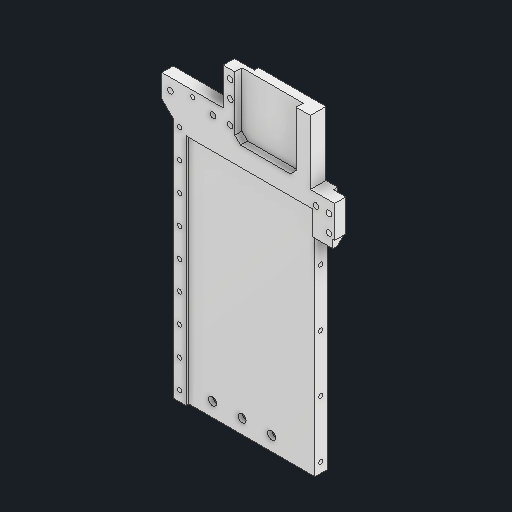
# Autodesk Inventor part: BottomSlideMount
Saved by Autodesk Inventor 2026.2 (Build 302298000, 298)
## iProperties
Created: 2026-01-21
Part Number: BottomSlideMount
Material: ABS Plastic
Document SubType Name: Modeling
Designer: gaoet
Density: 1.06 g/cm^3
Appearance: Smooth - White
Author: gaoet
Autodesk Inventor part; units mm, degrees
ref_plane "YZ Plane" through (0, 0, 0) normal (1, 0, 0) x (0, 1, 0)
ref_plane "XZ Plane" through (0, 0, 0) normal (0, 1, 0) x (-1, 0, 0)
ref_plane "XY Plane" through (0, 0, 0) normal (0, 0, 1) x (1, 0, 0)
sketch "Sketch1" plane through (0, 0, 0) normal (0, 0, 1) x (1, 0, 0)
  line L0 (-117.5, -110) -> (117.5, -110)
  line L1 (117.5, -110) -> (117.5, 110)
  line L2 (117.5, 110) -> (-117.5, 110)
  line L3 (-117.5, 110) -> (-117.5, -110)
  line L4 (-117.5, -110) -> (117.5, 110) construction
  line L5 (117.5, -110) -> (-117.5, 110) construction
  line L6 (0, 110) -> (0, -110) construction
  line L7 (-4, -110) -> (4, -110) construction
  line L8 (4, -110) -> (4, 110) construction
  line L9 (4, 110) -> (-4, 110) construction
  line L10 (-4, 110) -> (-4, -110) construction
  line L11 (-4, -110) -> (4, 110) construction
  line L12 (4, -110) -> (-4, 110) construction
  line L13 (-12, -110) -> (12, -110) construction
  line L14 (12, -110) -> (12, 110) construction
  line L15 (12, 110) -> (-12, 110) construction
  line L16 (-12, 110) -> (-12, -110) construction
  line L17 (-12, -110) -> (12, 110) construction
  line L18 (12, -110) -> (-12, 110) construction
  line L19 (-13, -110) -> (13, -110)
  line L20 (13, -110) -> (13, 110)
  line L21 (13, 110) -> (-13, 110)
  line L22 (-13, 110) -> (-13, -110)
  line L23 (-13, -110) -> (13, 110) construction
  line L24 (13, -110) -> (-13, 110) construction
  point P0 (0, 0)
  point P1 (-13, -110)
  point P2 (-13, 110)
  dimension "d0" = 235
  dimension "d1" = 220
  dimension "d4" = 8
  dimension "d5" = 24
  dimension "d6" = 26
  constraints: 50 end point, 10 midpoint, 8 parallel, 4 horizontal, 4 perpendicular, 3 point on line
  measures "d0" distance of L2.end L1.end
  measures "d1" distance of L1.end L0.end
  measures "d4" distance of L9.end L8.end
  measures "d5" distance of L15.end L14.end
  measures "d6" distance of L21.end L20.end
extrude "Extrusion1" add sketch "Sketch1" along normal blind 8 contours L3 L2 L22 L0
sketch "Sketch2" plane through (0, 0, 8) normal (0, 0, 1) x (1, 0, 0)
  line L0 (-13, 110) -> (-117.5, 110) projected
  line L1 (-13, -110) -> (-13, 110) projected
  point P0 (0, 0)
  point P1 (-17.25, 102)
  point P2 (-17.25, 90)
  dimension "d7" = 8
  dimension "d8" = 12
  dimension "d9" = 4.25
  constraints: 1 vertical alignment
  measures "d7" distance from line of L0 point (-17.25, 102)
  measures "d8" distance of point (-17.25, 90) point (-17.25, 102)
  measures "d9" distance from line of L1 point (-17.25, 90)
hole "Hole1" at (-17.25, 102, 8) direction (0, 0, -1) diameter 4 end through all
sketch "Sketch3" plane through (0, 0, 8) normal (0, 0, 1) x (1, 0, 0)
  line L0 (-117.5, -110) -> (-13, -110) projected
  line L1 (-13, -110) -> (-13, 110) projected
  line L2 (-13, 110) -> (-117.5, 110) projected
  line L3 (-117.5, 110) -> (-117.5, -110) projected
  line L4 (-13, 110) -> (-4.25, 110)
  line L5 (-4.25, 110) -> (-4.25, 82)
  line L6 (-4.25, 82) -> (-13, 82)
  line L7 (-13, 82) -> (-13, 110)
  point P0 (0, 0)
  point P1 (-13, 82)
  dimension "d17" = 8.75
  dimension "d18" = 28
  constraints: 8 end point, 2 parallel, 1 horizontal, 1 perpendicular
  measures "d17" distance of L5.end L6.end
  measures "d18" distance of L4.end L5.end
extrude "Extrusion2" add sketch "Sketch3" against normal up to surface (8 mm away) contours L1 L4 L5 L6
sketch "Sketch4" plane through (0, 0, 8) normal (0, 0, 1) x (1, 0, 0)
  circle A0 centre (-17.25, 102) radius 2 projected
  line L0 (-117.5, -110) -> (-13, -110) projected
  line L1 (-13, -110) -> (-13, 82) projected
  line L2 (-13, 82) -> (-4.25, 82) projected
  line L3 (-4.25, 82) -> (-4.25, 110) projected
  line L4 (-4.25, 110) -> (-117.5, 110) projected
  line L5 (-117.5, 110) -> (-117.5, -110) projected
  point P0 (0, 0)
  point P1 (-8.25, 102)
  point P2 (-8.25, 90)
  dimension "d21" = 4
  constraints: 1 horizontal alignment, 1 vertical alignment
  measures "d21" distance from line of L3 point (-8.25, 102)
hole "Hole2" at (-8.25, 102, 8) at (-8.25, 90, 8) direction (0, 0, -1) diameter 4 end through all
sketch "Sketch5" plane through (0, 0, 8) normal (0, 0, 1) x (1, 0, 0)
  circle A0 centre (-8.25, 90) radius 2 projected
  circle A1 centre (-8.25, 102) radius 2 projected
  circle A2 centre (-17.25, 102) radius 2 projected
  line L0 (-117.5, -110) -> (-13, -110) projected
  line L1 (-13, -110) -> (-13, 82) projected
  line L2 (-13, 82) -> (-4.25, 82) projected
  line L3 (-4.25, 82) -> (-4.25, 110) projected
  line L4 (-4.25, 110) -> (-117.5, 110) projected
  line L5 (-117.5, 110) -> (-117.5, -110) projected
  line L6 (-5.375, 82) -> (-5.375, 87.5)
  line L7 (-5.375, 87.5) -> (-4.25, 87.5)
  point P0 (0, 0)
  dimension "d29" = 5.5
  dimension "d30" = 1.125
  constraints: 4 end point, 2 point on line, 1 horizontal, 1 perpendicular
  measures "d29" distance of L6.start L6.end
  measures "d30" distance of L6.end L7.end
extrude "Extrusion3" cut sketch "Sketch5" against normal blind 10 contours L6 L7 L3 L2
sketch "Sketch6" plane through (-117.5, -110, 0) normal (0, -1, 0) x (1, 0, 0)
  line L0 (0, 0) -> (104.5, 0) projected
  line L1 (104.5, 0) -> (104.5, 8) projected
  line L2 (0, 8) -> (104.5, 8) projected
  line L3 (0, 0) -> (0, 8) projected
  line L4 (0, 0) -> (0, 8) projected
  line L5 (0, 5) -> (15.25, 5)
  line L6 (15.25, 5) -> (15.25, 0)
  line L7 (9, 5) -> (9, 3.5)
  line L8 (9, 3.5) -> (15.25, 3.5)
  point P0 (117.5, 0)
  point P1 (0, 4)
  dimension "d33" = 15.25
  dimension "d34" = 5
  dimension "d35" = 9
  dimension "d36" = 1.5
  constraints: 8 end point, 4 point on line, 2 perpendicular, 1 horizontal, 1 midpoint, 1 vertical
  measures "d33" distance of L5.start L5.end
  measures "d34" distance of L5.end L6.end
  measures "d35" distance from line of point (0, 4) L7
  measures "d36" distance between parallel lines of L5 L8
extrude "Extrusion4" cut sketch "Sketch6" against normal through all contours L3 L5 L7 L8 L6 L0
chamfer "Chamfer1" distance 5 angle 45 1 edges at (-9.1875, 82, 0)
sketch "Sketch7" plane through (0, 0, 8) normal (0, 0, 1) x (1, 0, 0)
  line L0 (-117.5, -65) -> (-13, -65)
  line L1 (-5.375, 87.5) -> (-4.25, 87.5) projected
  line L2 (-4.25, 87.5) -> (-4.25, 110) projected
  line L3 (-4.25, 110) -> (-117.5, 110) projected
  line L4 (-117.5, 110) -> (-117.5, -110) projected
  line L5 (-117.5, -110) -> (-13, -110) projected
  line L6 (-13, -110) -> (-13, 82) projected
  line L7 (-13, 82) -> (-5.375, 82) projected
  line L8 (-5.375, 82) -> (-5.375, 87.5) projected
  circle A0 centre (-8.25, 90) radius 2 projected
  circle A1 centre (-8.25, 102) radius 2 projected
  circle A2 centre (-17.25, 102) radius 2 projected
  point P0 (0, 0)
  dimension "d42" = 45
  constraints: 2 end point, 2 point on line, 1 horizontal, 1 perpendicular
  measures "d42" distance between parallel lines of L5 L0
extrude "Extrusion5" cut sketch "Sketch7" against normal blind 10 contours L0 L6 L5 L4
sketch "Sketch8" plane through (-117.5, 110, 8) normal (0, 1, 0) x (1, 0, 0)
  line L0 (113.25, 0) -> (0, 0) projected
  line L1 (15.25, 8) -> (15.25, 4.5) projected
  line L2 (15.25, 4.5) -> (9, 4.5) projected
  line L3 (9, 4.5) -> (9, 3) projected
  line L4 (9, 3) -> (0, 3) projected
  line L5 (0, 3) -> (0, 0) projected
  line L6 (113.25, 0) -> (0, 0) projected
  line L7 (113.25, 0) -> (113.25, 8) projected
  line L8 (15.25, 8) -> (113.25, 8) projected
  line L9 (96.25, 0) -> (96.25, 8)
  line L10 (15.25, 8) -> (0, 8)
  line L11 (0, 8) -> (0, 3)
  point P0 (117.5, 8)
  point P1 (96.25, 4)
  dimension "d45" = 96.25
  constraints: 6 end point, 2 perpendicular, 2 point on line, 1 horizontal, 1 midpoint
  measures "d45" horizontal distance of L4.end point (96.25, 4)
extrude "Extrusion6" add sketch "Sketch8" along normal blind 45 contours L0 L5 L4 L3 L2 L1 L8 L9 | L11 L10 L1 L2 L3 L4
sketch "Sketch9" plane through (0, 0, 0) normal (0, 0, -1) x (-1, 0, 0)
  line L0 (13, -65) -> (102.25, -65) projected
  line L1 (102.25, -65) -> (102.25, 110) projected
  line L2 (102.25, 110) -> (117.5, 110) projected
  line L3 (117.5, 110) -> (117.5, 155) projected
  line L4 (21.25, 155) -> (117.5, 155) projected
  line L5 (21.25, 110) -> (21.25, 155) projected
  line L6 (21.25, 110) -> (4.25, 110) projected
  line L7 (4.25, 110) -> (4.25, 87.5) projected
  line L8 (4.25, 87.5) -> (5.375, 87.5) projected
  line L9 (5.375, 87.5) -> (5.375, 87) projected
  line L10 (13, 87) -> (5.375, 87) projected
  line L11 (13, -65) -> (13, 87) projected
  circle A0 centre (8.25, 90) radius 2 projected
  circle A1 centre (8.25, 102) radius 2 projected
  circle A2 centre (17.25, 102) radius 2 projected
  line L12 (82.5, 155) -> (82.5, 129)
  line L13 (82.5, 129) -> (117.5, 129)
  line L14 (21.25, 155) -> (117.5, 155) projected
  point P0 (0, 0)
  dimension "d49" = 35
  dimension "d50" = 26
  constraints: 4 end point, 2 point on line, 1 perpendicular, 1 vertical
  measures "d49" distance of L12.end L13.end
  measures "d50" distance of L12.start L12.end
extrude "Extrusion7" cut sketch "Sketch9" against normal through all contours L13 L12 L4 L3
sketch "Sketch10" plane through (0, 0, 0) normal (0, 0, -1) x (-1, 0, 0)
  line L0 (21.25, 155) -> (82.5, 155) projected
  line L1 (82.5, 129) -> (82.5, 155) projected
  point P0 (0, 0)
  point P1 (77.5, 149)
  point P2 (77.5, 137)
  point P3 (77.5, 121)
  point P4 (89.5, 121)
  point P5 (119.5, 121)
  dimension "d53" = 12
  dimension "d54" = 6
  dimension "d55" = 16
  dimension "d56" = 5
  dimension "d57" = 12
  dimension "d58" = 30
  constraints: 2 horizontal alignment, 2 vertical alignment
  measures "d53" distance of point (77.5, 149) point (77.5, 137)
  measures "d54" distance from line of L0 point (77.5, 149)
  measures "d55" distance of point (77.5, 137) point (77.5, 121)
  measures "d56" distance from line of point (77.5, 149) L1
  measures "d57" distance of point (89.5, 121) point (77.5, 121)
  measures "d58" distance of point (89.5, 121) point (119.5, 121)
sketch "Sketch11" plane through (-117.5, 110, 8) normal (0, -1, 0) x (1, 0, 0)
  line L0 (15.25, -8) -> (15.25, -4.5) projected
  line L1 (15.25, -4.5) -> (9, -4.5) projected
  line L2 (9, -4.5) -> (9, -3) projected
  line L3 (9, -3) -> (0, -3) projected
  line L4 (0, -8) -> (0, -3) projected
  line L5 (15.25, -8) -> (0, -8) projected
  point P0 (117.5, -8)
extrude "Extrusion8" add sketch "Sketch11" along normal blind 26
sketch "Sketch12" plane through (0, 0, 0) normal (0, 0, -1) x (-1, 0, 0)
  line L0 (82.5, 129) -> (82.5, 155) projected
  line L1 (21.25, 155) -> (82.5, 155) projected
  line L2 (21.25, 110) -> (21.25, 155) projected
  line L3 (21.25, 110) -> (4.25, 110) projected
  line L4 (4.25, 110) -> (4.25, 87.5) projected
  line L5 (4.25, 87.5) -> (5.375, 87.5) projected
  line L6 (5.375, 87.5) -> (5.375, 87) projected
  line L7 (13, 87) -> (5.375, 87) projected
  line L8 (13, -65) -> (13, 87) projected
  line L9 (13, -65) -> (102.25, -65) projected
  line L10 (102.25, -65) -> (102.25, 84) projected
  line L11 (117.5, 84) -> (102.25, 84) projected
  line L12 (117.5, 129) -> (117.5, 84) projected
  line L13 (117.5, 129) -> (82.5, 129) projected
  circle A0 centre (8.25, 90) radius 2 projected
  circle A1 centre (8.25, 102) radius 2 projected
  circle A2 centre (17.25, 102) radius 2 projected
  line L14 (117.5, 129) -> (125.5, 129)
  line L15 (125.5, 129) -> (125.5, 113)
  line L16 (125.5, 113) -> (117.5, 113)
  point P0 (0, 0)
  point P1 (125.5, 121)
  dimension "d61" = 8
  dimension "d62" = 16
  constraints: 6 end point, 2 horizontal, 1 midpoint, 1 perpendicular, 1 point on line
  measures "d61" distance from line of L12 point (125.5, 121)
  measures "d62" distance of L14.end L15.end
extrude "Extrusion9" add sketch "Sketch12" against normal up to surface (8 mm away) contours L14 L15 L16 L12
chamfer "Chamfer2" distance 8 angle 45 1 edges at (-117.5, 113, 4)
hole "Hole3" at (-77.5, 149, 0) at (-77.5, 137, 0) at (-77.5, 121, 0) at (-89.5, 121, 0) at (-119.5, 121, 0) direction (0, 0, 1) diameter 4 end through all
sketch "Sketch13" plane through (0, 0, 0) normal (0, 0, -1) x (-1, 0, 0)
  line L0 (117.5, 105) -> (117.5, 84) projected
  line L1 (125.5, 129) -> (82.5, 129) projected
  point P0 (0, 0)
  point P1 (103.75, 125)
  dimension "d75" = 13.75
  dimension "d76" = 4
  measures "d75" distance from line of L0 point (103.75, 125)
  measures "d76" distance from line of L1 point (103.75, 125)
hole "Hole4" at (-103.75, 125, 0) direction (0, 0, 1) diameter 3 end through all
sketch "Sketch14" plane through (0, 0, 0) normal (0, 0, -1) x (-1, 0, 0)
  circle A0 centre (103.75, 125) radius 1.5 projected
  circle A1 centre (119.5, 121) radius 2 projected
  circle A2 centre (89.5, 121) radius 2 projected
  circle A3 centre (77.5, 121) radius 2 projected
  circle A4 centre (77.5, 137) radius 2 projected
  circle A5 centre (77.5, 149) radius 2 projected
  line L0 (82.5, 129) -> (82.5, 155) projected
  line L1 (21.25, 155) -> (82.5, 155) projected
  line L2 (21.25, 110) -> (21.25, 155) projected
  line L3 (21.25, 110) -> (4.25, 110) projected
  line L4 (4.25, 110) -> (4.25, 87.5) projected
  line L5 (4.25, 87.5) -> (5.375, 87.5) projected
  line L6 (5.375, 87.5) -> (5.375, 87) projected
  line L7 (13, 87) -> (5.375, 87) projected
  line L8 (13, -65) -> (13, 87) projected
  line L9 (13, -65) -> (102.25, -65) projected
  line L10 (102.25, -65) -> (102.25, 84) projected
  line L11 (117.5, 84) -> (102.25, 84) projected
  line L12 (117.5, 105) -> (117.5, 84) projected
  line L13 (125.5, 113) -> (117.5, 105) projected
  line L14 (125.5, 113) -> (125.5, 129) projected
  line L15 (125.5, 129) -> (82.5, 129) projected
  circle A6 centre (8.25, 90) radius 2 projected
  circle A7 centre (8.25, 102) radius 2 projected
  circle A8 centre (17.25, 102) radius 2 projected
  line L16 (105.3233, 127.725) -> (106.8966, 125)
  line L17 (106.8966, 125) -> (105.3233, 122.275)
  line L18 (105.3233, 122.275) -> (102.1767, 122.275)
  line L19 (102.1767, 122.275) -> (100.6034, 125)
  line L20 (100.6034, 125) -> (102.1767, 127.725)
  line L21 (102.1767, 127.725) -> (105.3233, 127.725)
  point P0 (0, 0)
  point P1 (103.75, 122.275)
  dimension "d84" = 5.45
  constraints: 12 end point, 1 coincident, 1 horizontal, 1 midpoint, 13 other
  measures "d84" distance from line of point (103.75, 122.275) L21
extrude "Extrusion10" cut sketch "Sketch14" against normal blind 2.5 contours L16 L17 L18 L19 L20 L21
sketch "Sketch15" plane through (-117.5, 84, 8) normal (0, -1, 0) x (1, 0, 0)
  line L0 (15.25, -4.5) -> (15.25, -8) projected
  line L1 (9, -4.5) -> (15.25, -4.5) projected
  line L2 (9, -3) -> (9, -4.5) projected
  line L3 (0, -3) -> (9, -3) projected
  line L4 (0, -3) -> (0, -8) projected
  line L5 (0, -8) -> (15.25, -8) projected
  point P0 (117.5, -8)
extrude "Extrusion11" cut sketch "Sketch15" against normal blind 23
sketch "Sketch16" plane through (-108.5, -65, 5) normal (0, 0, -1) x (-1, 0, 0)
  line L0 (9, 172) -> (9, 170) projected
  line L1 (0, 0) -> (0, 172) projected
  line L2 (-6.25, 172) -> (9, 172) projected
  line L3 (9, 170) -> (9, 0) projected
  point P0 (-108.5, 65)
  point P1 (4.5, 167)
  point P2 (4.5, 147)
  point P3 (4.5, 127)
  point P4 (4.5, 107)
  point P5 (4.5, 87)
  point P6 (4.5, 67)
  point P7 (4.5, 47)
  point P8 (4.5, 27)
  point P9 (4.5, 7)
  point P10 (4.5, -13)
  point P11 (4.5, -33)
  dimension "d89" = 9
  dimension "d90" = 5
  dimension "d91" = 4.5
  dimension "d94" = 20
  constraints: 1 vertical, 10 other
  measures "d89" distance between parallel lines of L0 L1
  measures "d90" distance from line of L2 point (4.5, 167)
  measures "d91" distance from line of L3 point (4.5, 167)
  measures "d94" distance of point (4.5, 167) point (4.5, 147)
hole "Hole5" at (-113, 102, 5) at (-113, 82, 5) at (-113, 62, 5) at (-113, 42, 5) at (-113, 22, 5) at (-113, 2, 5) at (-113, -18, 5) at (-113, -38, 5) at (-113, -58, 5) at (-113, -78, 5) at (-113, -98, 5) direction (0, 0, 1) diameter 3 depth 12
sketch "Sketch17" plane through (0, 0, 8) normal (0, 0, 1) x (1, 0, 0)
  circle A0 centre (-113, -58) radius 1.5 projected
  circle A1 centre (-113, -38) radius 1.5 projected
  circle A2 centre (-113, -18) radius 1.5 projected
  circle A3 centre (-113, 2) radius 1.5 projected
  circle A4 centre (-113, 22) radius 1.5 projected
  circle A5 centre (-113, 42) radius 1.5 projected
  circle A6 centre (-113, 62) radius 1.5 projected
  circle A7 centre (-113, 82) radius 1.5 projected
  circle A8 centre (-113, 102) radius 1.5 projected
  circle A9 centre (-103.75, 125) radius 1.5 projected
  circle A10 centre (-119.5, 121) radius 2 projected
  circle A11 centre (-89.5, 121) radius 2 projected
  circle A12 centre (-77.5, 121) radius 2 projected
  circle A13 centre (-77.5, 137) radius 2 projected
  circle A14 centre (-77.5, 149) radius 2 projected
  line L0 (-82.5, 155) -> (-82.5, 129) projected
  line L1 (-82.5, 129) -> (-125.5, 129) projected
  line L2 (-125.5, 113) -> (-125.5, 129) projected
  line L3 (-117.5, 105) -> (-125.5, 113) projected
  line L4 (-117.5, -65) -> (-117.5, 105) projected
  line L5 (-117.5, -65) -> (-13, -65) projected
  line L6 (-13, -65) -> (-13, 82) projected
  line L7 (-13, 82) -> (-5.375, 82) projected
  line L8 (-5.375, 82) -> (-5.375, 87.5) projected
  line L9 (-5.375, 87.5) -> (-4.25, 87.5) projected
  line L10 (-4.25, 87.5) -> (-4.25, 110) projected
  line L11 (-4.25, 110) -> (-21.25, 110) projected
  line L12 (-21.25, 110) -> (-21.25, 155) projected
  line L13 (-82.5, 155) -> (-21.25, 155) projected
  circle A15 centre (-8.25, 90) radius 2 projected
  circle A16 centre (-8.25, 102) radius 2 projected
  circle A17 centre (-17.25, 102) radius 2 projected
  line L14 (-13, 82) -> (-20, 82)
  line L15 (-20, 82) -> (-20, -65)
  line L16 (-20, -65) -> (-13, -65)
  line L17 (-13, -65) -> (-13, 82)
  point P0 (0, 0)
  dimension "d106" = 7
  constraints: 8 end point, 2 parallel, 1 horizontal, 1 perpendicular, 1 point on line
  measures "d106" distance between parallel lines of L6 L15
extrude "Extrusion12" cut sketch "Sketch17" against normal blind 10 contours L15 L14 L6 L5
sketch "Sketch18" plane through (0, 0, 0) normal (0, 0, -1) x (-1, 0, 0)
  circle A0 centre (17.25, 102) radius 2 projected
  circle A1 centre (8.25, 102) radius 2 projected
  circle A2 centre (8.25, 90) radius 2 projected
  circle A3 centre (77.5, 149) radius 2 projected
  circle A4 centre (77.5, 137) radius 2 projected
  circle A5 centre (77.5, 121) radius 2 projected
  circle A6 centre (89.5, 121) radius 2 projected
  circle A7 centre (119.5, 121) radius 2 projected
  line L0 (102.1767, 122.275) -> (100.6034, 125) projected
  line L1 (100.6034, 125) -> (102.1767, 127.725) projected
  line L2 (102.1767, 127.725) -> (105.3233, 127.725) projected
  line L3 (105.3233, 127.725) -> (106.8966, 125) projected
  line L4 (106.8966, 125) -> (105.3233, 122.275) projected
  line L5 (105.3233, 122.275) -> (102.1767, 122.275) projected
  line L6 (13, 82) -> (20, 82) projected
  line L7 (20, 82) -> (20, -65) projected
  line L8 (20, -65) -> (102.25, -65) projected
  line L9 (102.25, -65) -> (102.25, 107) projected
  line L10 (102.25, 107) -> (117.5, 107) projected
  line L11 (117.5, 107) -> (117.5, 105) projected
  line L12 (125.5, 113) -> (117.5, 105) projected
  line L13 (125.5, 113) -> (125.5, 129) projected
  line L14 (125.5, 129) -> (82.5, 129) projected
  line L15 (82.5, 129) -> (82.5, 155) projected
  line L16 (21.25, 155) -> (82.5, 155) projected
  line L17 (21.25, 110) -> (21.25, 155) projected
  line L18 (21.25, 110) -> (4.25, 110) projected
  line L19 (4.25, 110) -> (4.25, 87.5) projected
  line L20 (4.25, 87.5) -> (5.375, 87.5) projected
  line L21 (5.375, 87.5) -> (5.375, 87) projected
  line L22 (13, 87) -> (5.375, 87) projected
  line L23 (13, 82) -> (13, 87) projected
  line L24 (125.5, 155) -> (68.5, 155)
  line L25 (68.5, 155) -> (68.5, 116)
  line L26 (68.5, 116) -> (125.5, 116)
  line L27 (125.5, 116) -> (125.5, 155)
  line L28 (21.25, 155) -> (82.5, 155) projected
  line L29 (125.5, 113) -> (125.5, 129) projected
  line L30 (13, 82) -> (13, 87) projected
  line L31 (13, 87) -> (13, 110)
  point P0 (0, 0)
  point P1 (125.5, 129)
  dimension "d109" = 14
  dimension "d110" = 39
  constraints: 10 end point, 2 collinear, 2 parallel, 1 horizontal, 1 perpendicular, 1 point on line, 1 vertical
  measures "d109" distance between parallel lines of L15 L25
  measures "d110" distance between parallel lines of L16 L26
extrude "Extrusion13" add sketch "Sketch18" along normal blind 3 contours L23 L31 L18 L17 L16 L25 L26 L13 L12 L11 L10 L9 L8 L7 L6
sketch "Sketch19" plane through (-20, -65, 8) normal (1, 0, 0) x (0, 0, -1)
  line L0 (11, 0) -> (0, 0) projected
  line L1 (11, 147) -> (11, 0) projected
  point P0 (8, 65)
  point P1 (6, -33)
  point P2 (6, 7)
  point P3 (6, 47)
  point P4 (6, 127)
  point P5 (6, 87)
  dimension "d113" = 40
  dimension "d114" = 7
  dimension "d115" = 40
  dimension "d116" = 40
  dimension "d117" = 40
  dimension "d118" = 5
  constraints: 4 vertical alignment
  measures "d113" distance of point (6, 7) point (6, -33)
  measures "d114" distance from line of L0 point (6, 7)
  measures "d115" distance of point (6, 47) point (6, 7)
  measures "d116" distance of point (6, 87) point (6, 47)
  measures "d117" distance of point (6, 127) point (6, 87)
  measures "d118" distance from line of L1 point (6, 7)
hole "Hole6" at (-20, -98, 2) at (-20, -58, 2) at (-20, -18, 2) at (-20, 62, 2) at (-20, 22, 2) direction (-1, 0, 0) diameter 3 depth 15
sketch "Sketch20" plane through (0, 0, -3) normal (0, 0, -1) x (-1, 0, 0)
  line L0 (117.5, 105) -> (125.5, 113) projected
  line L1 (125.5, 113) -> (125.5, 116) projected
  line L2 (125.5, 116) -> (68.5, 116) projected
  line L3 (68.5, 116) -> (68.5, 155) projected
  line L4 (68.5, 155) -> (21.25, 155) projected
  line L5 (21.25, 155) -> (21.25, 110) projected
  line L6 (21.25, 110) -> (13, 110) projected
  line L7 (13, 110) -> (13, 82) projected
  line L8 (13, 82) -> (20, 82) projected
  line L9 (20, 82) -> (20, -65) projected
  line L10 (20, -65) -> (102.25, -65) projected
  line L11 (102.25, -65) -> (102.25, 107) projected
  line L12 (102.25, 107) -> (117.5, 107) projected
  line L13 (117.5, 107) -> (117.5, 105) projected
  circle A0 centre (17.25, 102) radius 2 projected
  line L14 (102.25, -45) -> (20, -45)
  line L15 (35, -56.5) -> (35, -59.5) projected
  line L16 (40, -65) -> (40, -45)
  point P0 (0, 0)
  dimension "d126" = 20
  dimension "d127" = 20
  constraints: 4 end point, 4 point on line, 1 horizontal, 1 perpendicular
  measures "d126" distance between parallel lines of L10 L14
  measures "d127" distance between parallel lines of L9 L16
extrude "Extrusion14" cut sketch "Sketch20" against normal blind 3.5 contours L11 L10 L16 L14
chamfer "Chamfer3" distance 10 angle 45 2 edges at (-40, -45, -1.25) (-40, -65, -1.25)
sketch "Sketch21" plane through (0, 0, 8) normal (0, 0, 1) x (1, 0, 0)
  line L0 (-50, -45) -> (-30, -65) projected
  line L1 (-102.25, -65) -> (-30, -65) projected
  line L2 (-102.25, -45) -> (-102.25, -65) projected
  line L3 (-50, -45) -> (-102.25, -45) projected
  point P0 (0, 0)
  point P1 (-91.875, -55)
  point P2 (-71.125, -55)
  point P3 (-50.375, -55)
  point P4 (-102.25, -55)
  dimension "d133" = 20
  dimension "d134" = 20.75
  dimension "d135" = 20.75
  dimension "d136" = 10.375
  dimension "d137" = 10
  constraints: 2 horizontal alignment, 1 midpoint
  measures "d133" distance between parallel lines of L1 L3
  measures "d134" distance of point (-91.875, -55) point (-71.125, -55)
  measures "d135" distance of point (-50.375, -55) point (-71.125, -55)
  measures "d136" distance of point (-102.25, -55) point (-91.875, -55)
  measures "d137" distance from line of L1 point (-91.875, -55)
hole "Hole7" at (-91.875, -55, 8) at (-71.125, -55, 8) at (-50.375, -55, 8) direction (0, 0, -1) diameter 3 depth 15 counterbore diameter 5.75 counterbore depth 5
sketch "Sketch22" plane through (0, 0, 8) normal (0, 0, 1) x (1, 0, 0)
  circle A0 centre (-50.375, -55) radius 2.875 projected
  circle A1 centre (-71.125, -55) radius 2.875 projected
  circle A2 centre (-91.875, -55) radius 2.875 projected
  line L0 (-20, 82) -> (-5.375, 82) projected
  line L1 (-5.375, 82) -> (-5.375, 87.5) projected
  line L2 (-5.375, 87.5) -> (-4.25, 87.5) projected
  line L3 (-4.25, 87.5) -> (-4.25, 110) projected
  line L4 (-4.25, 110) -> (-21.25, 110) projected
  line L5 (-21.25, 110) -> (-21.25, 155) projected
  line L6 (-82.5, 155) -> (-21.25, 155) projected
  line L7 (-82.5, 155) -> (-82.5, 129) projected
  line L8 (-82.5, 129) -> (-125.5, 129) projected
  line L9 (-125.5, 113) -> (-125.5, 129) projected
  line L10 (-117.5, 105) -> (-125.5, 113) projected
  line L11 (-117.5, -65) -> (-117.5, 105) projected
  line L12 (-117.5, -65) -> (-20, -65) projected
  line L13 (-20, -65) -> (-20, 82) projected
  circle A3 centre (-113, -58) radius 1.5 projected
  circle A4 centre (-113, -38) radius 1.5 projected
  circle A5 centre (-113, -18) radius 1.5 projected
  circle A6 centre (-113, 2) radius 1.5 projected
  circle A7 centre (-113, 22) radius 1.5 projected
  circle A8 centre (-113, 42) radius 1.5 projected
  circle A9 centre (-113, 62) radius 1.5 projected
  circle A10 centre (-113, 82) radius 1.5 projected
  circle A11 centre (-113, 102) radius 1.5 projected
  circle A12 centre (-103.75, 125) radius 1.5 projected
  circle A13 centre (-119.5, 121) radius 2 projected
  circle A14 centre (-89.5, 121) radius 2 projected
  circle A15 centre (-77.5, 121) radius 2 projected
  circle A16 centre (-77.5, 137) radius 2 projected
  circle A17 centre (-77.5, 149) radius 2 projected
  circle A18 centre (-8.25, 90) radius 2 projected
  circle A19 centre (-8.25, 102) radius 2 projected
  circle A20 centre (-17.25, 102) radius 2 projected
  line L14 (-117.5, 99) -> (-20, 99)
  line L15 (-20, 82) -> (-20, 110)
  line L16 (-108.5, 99) -> (-108.5, -65)
  point P0 (0, 0)
  point P1 (-20, 99)
  dimension "d145" = 56
  dimension "d146" = 9
  constraints: 6 end point, 5 point on line, 2 vertical, 1 perpendicular
  measures "d145" distance between parallel lines of L6 L14
  measures "d146" distance between parallel lines of L11 L16
extrude "Extrusion15" cut sketch "Sketch22" against normal blind 2 contours L13 L12 L16 L14 L15
sketch "Sketch23" plane through (0, 0, 8) normal (0, 0, 1) x (1, 0, 0)
  line L0 (-31.75, 155) -> (-73.75, 155)
  line L1 (-73.75, 155) -> (-73.75, 113)
  line L2 (-73.75, 113) -> (-31.75, 113)
  line L3 (-31.75, 113) -> (-31.75, 155)
  line L4 (-31.75, 155) -> (-73.75, 113) construction
  line L5 (-73.75, 155) -> (-31.75, 113) construction
  line L6 (-82.5, 155) -> (-82.5, 129) projected
  line L7 (-82.5, 155) -> (-21.25, 155) projected
  circle A0 centre (-17.25, 102) radius 2 projected
  circle A1 centre (-8.25, 102) radius 2 projected
  circle A2 centre (-8.25, 90) radius 2 projected
  circle A3 centre (-77.5, 149) radius 2 projected
  circle A4 centre (-77.5, 137) radius 2 projected
  circle A5 centre (-77.5, 121) radius 2 projected
  circle A6 centre (-89.5, 121) radius 2 projected
  circle A7 centre (-119.5, 121) radius 2 projected
  circle A8 centre (-103.75, 125) radius 1.5 projected
  circle A9 centre (-113, 102) radius 1.5 projected
  circle A10 centre (-113, 82) radius 1.5 projected
  circle A11 centre (-113, 62) radius 1.5 projected
  circle A12 centre (-113, 42) radius 1.5 projected
  circle A13 centre (-113, 22) radius 1.5 projected
  circle A14 centre (-113, 2) radius 1.5 projected
  circle A15 centre (-113, -18) radius 1.5 projected
  circle A16 centre (-113, -38) radius 1.5 projected
  circle A17 centre (-113, -58) radius 1.5 projected
  line L8 (-108.5, -65) -> (-108.5, 99) projected
  line L9 (-108.5, 99) -> (-20, 99) projected
  line L10 (-20, 99) -> (-20, 82) projected
  line L11 (-20, 82) -> (-5.375, 82) projected
  line L12 (-5.375, 82) -> (-5.375, 87.5) projected
  line L13 (-5.375, 87.5) -> (-4.25, 87.5) projected
  line L14 (-4.25, 87.5) -> (-4.25, 110) projected
  line L15 (-4.25, 110) -> (-21.25, 110) projected
  line L16 (-21.25, 110) -> (-21.25, 155) projected
  line L17 (-82.5, 155) -> (-21.25, 155) projected
  line L18 (-82.5, 155) -> (-82.5, 129) projected
  line L19 (-82.5, 129) -> (-125.5, 129) projected
  line L20 (-125.5, 113) -> (-125.5, 129) projected
  line L21 (-117.5, 105) -> (-125.5, 113) projected
  line L22 (-117.5, -65) -> (-117.5, 105) projected
  line L23 (-117.5, -65) -> (-108.5, -65) projected
  line L24 (-31.25, 112.5) -> (-74.25, 112.5)
  line L25 (-74.25, 112.5) -> (-74.25, 155.5)
  line L26 (-74.25, 155.5) -> (-31.25, 155.5)
  line L27 (-31.25, 155.5) -> (-31.25, 112.5)
  point P0 (0, 0)
  point P1 (-52.75, 134)
  dimension "d149" = 42
  dimension "d150" = 42
  dimension "d151" = 8.75
  dimension "d152" = 0.5
  constraints: 20 end point, 4 parallel, 2 midpoint, 2 perpendicular, 1 collinear, 1 horizontal, 3 other
  measures "d149" distance of L2.end L1.end
  measures "d150" distance of L1.end L0.end
  measures "d151" distance between parallel lines of L6 L1
  measures "d152" distance between parallel lines of L2 L24
extrude "Extrusion16" cut sketch "Sketch23" against normal blind 5 contours L3 L2 L1 L0 | L7 L27 L24 L25 L1 L2 L3 | L0 L7 L25 L26 L27
chamfer "Chamfer4" distance 4 angle 45 2 edges at (-31.25, 112.5, 5.5) (-74.25, 112.5, 5.5)
equation "\"d91\" = 0.5 * d89"
equation "\"d115\" = d113"
equation "\"d116\" = d115"
equation "\"d117\" = d116"
equation "\"d135\" = d134"
equation "\"d136\" = 0.5 * d134"
equation "\"d137\" = 0.5 * d133"
body "Solid1"
